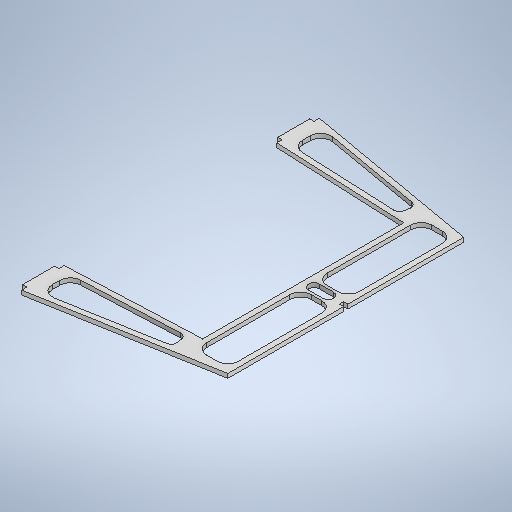
# Autodesk Inventor part: crush zone
Saved by Autodesk Inventor 2025.2 (Build 292293000, 293)
## iProperties
Created: 2025-01-25
Part Number: crush zone
Material: Generic
Document SubType Name: Modeling
Designer: alex
Density: 1 g/cm^3
Appearance: Default
Author: alex
Autodesk Inventor part; units mm, degrees
ref_plane "YZ Plane" through (0, 0, 0) normal (1, 0, 0) x (0, 1, 0)
ref_plane "XZ Plane" through (0, 0, 0) normal (0, 1, 0) x (-1, 0, 0)
ref_plane "XY Plane" through (0, 0, 0) normal (0, 0, 1) x (1, 0, 0)
sketch "Sketch1" plane through (0, 0, 0) normal (0, 1, 0) x (-1, 0, 0)
  line L0 (0, 0) -> (0, -76.2)
  line L1 (0, -76.2) -> (-10.16, -76.2)
  line L2 (-10.16, -76.2) -> (-10.16, -88.9)
  line L3 (-10.16, -88.9) -> (-327.3578, -102.7492)
  line L4 (0, 0) -> (-10.16, 0)
  line L5 (-10.16, 0) -> (-10.16, 12.7)
  line L6 (-10.16, 12.7) -> (-428.9578, -61.1454)
  line L7 (-428.9578, -61.1454) -> (-428.9578, -342.9)
  line L8 (-428.9578, -342.9) -> (-327.3578, -342.9)
  line L9 (-327.3578, -342.9) -> (-327.3578, -102.7492)
  line L10 (-365.4578, -323.85) -> (-390.8578, -323.85)
  line L11 (-416.2578, -298.45) -> (-416.2578, -99.2454)
  line L12 (-390.8578, -73.8454) -> (-365.4578, -73.8454)
  line L13 (-340.0578, -99.2454) -> (-340.0578, -298.45)
  line L14 (-294.1616, -50.2731) -> (-65.3707, -9.931)
  line L15 (-35.56, -34.9452) -> (-35.56, -52.9817)
  line L16 (-59.8521, -78.3575) -> (-289.4473, -88.3818)
  arc A0 (-340.0578, -99.2454) -> (-365.4578, -73.8454) centre (-365.4578, -99.2454) ccw
  arc A1 (-390.8578, -73.8454) -> (-416.2578, -99.2454) centre (-390.8578, -99.2454) ccw
  arc A2 (-416.2578, -298.45) -> (-390.8578, -323.85) centre (-390.8578, -298.45) ccw
  arc A3 (-365.4578, -323.85) -> (-340.0578, -298.45) centre (-365.4578, -298.45) ccw
  arc A4 (-35.56, -34.9452) -> (-65.3707, -9.931) centre (-60.96, -34.9452) ccw
  arc A5 (-59.8521, -78.3575) -> (-35.56, -52.9817) centre (-60.96, -52.9817) ccw
  line L17 (0, -685.8) -> (0, -609.6)
  line L18 (0, -609.6) -> (-10.16, -609.6)
  line L19 (-10.16, -609.6) -> (-10.16, -596.9)
  line L20 (-10.16, -596.9) -> (-327.3578, -583.0508)
  line L21 (0, -685.8) -> (-10.16, -685.8)
  line L22 (-10.16, -685.8) -> (-10.16, -698.5)
  line L23 (-10.16, -698.5) -> (-428.9578, -624.6546)
  line L24 (-428.9578, -624.6546) -> (-428.9578, -342.9)
  line L25 (-327.3578, -342.9) -> (-327.3578, -583.0508)
  line L26 (-365.4578, -361.95) -> (-390.8578, -361.95)
  line L27 (-416.2578, -387.35) -> (-416.2578, -586.5546)
  line L28 (-390.8578, -611.9546) -> (-365.4578, -611.9546)
  line L29 (-340.0578, -586.5546) -> (-340.0578, -387.35)
  line L30 (-294.1616, -635.5269) -> (-65.3707, -675.869)
  line L31 (-35.56, -650.8548) -> (-35.56, -632.8183)
  line L32 (-59.8521, -607.4425) -> (-289.4473, -597.4182)
  arc A6 (-365.4578, -611.9546) -> (-340.0578, -586.5546) centre (-365.4578, -586.5546) ccw
  arc A7 (-416.2578, -586.5546) -> (-390.8578, -611.9546) centre (-390.8578, -586.5546) ccw
  arc A8 (-390.8578, -361.95) -> (-416.2578, -387.35) centre (-390.8578, -387.35) ccw
  arc A9 (-340.0578, -387.35) -> (-365.4578, -361.95) centre (-365.4578, -387.35) ccw
  arc A10 (-65.3707, -675.869) -> (-35.56, -650.8548) centre (-60.96, -650.8548) ccw
  arc A11 (-35.56, -632.8183) -> (-59.8521, -607.4425) centre (-60.96, -632.8183) ccw
  line L33 (-428.9578, -337.82) -> (-418.7978, -337.82)
  line L34 (-418.7978, -337.82) -> (-418.7978, -347.98)
  line L35 (-418.7978, -347.98) -> (-428.9578, -347.98)
  line L36 (-387.0478, -330.2) -> (-352.7578, -330.2)
  line L37 (-340.0578, -342.9) -> (-340.0578, -342.9)
  line L38 (-352.7578, -355.6) -> (-387.0478, -355.6)
  line L39 (-399.7478, -342.9) -> (-399.7478, -342.9)
  arc A12 (-340.0578, -342.9) -> (-352.7578, -330.2) centre (-352.7578, -342.9) ccw
  arc A13 (-352.7578, -355.6) -> (-340.0578, -342.9) centre (-352.7578, -342.9) ccw
  arc A14 (-399.7478, -342.9) -> (-387.0478, -355.6) centre (-387.0478, -342.9) ccw
  arc A15 (-387.0478, -330.2) -> (-399.7478, -342.9) centre (-387.0478, -342.9) ccw
  line L40 (-304.5132, -64.681) -> (-302.5582, -77.5949)
  arc A16 (-294.1616, -50.2731) -> (-304.5132, -64.681) centre (-291.9562, -62.7801) ccw
  arc A17 (-302.5582, -77.5949) -> (-289.4473, -88.3818) centre (-290.0013, -75.6939) ccw
  line L41 (-304.5132, -621.119) -> (-302.5582, -608.2051)
  arc A18 (-289.4473, -597.4182) -> (-302.5582, -608.2051) centre (-290.0013, -610.1061) ccw
  arc A19 (-304.5132, -621.119) -> (-294.1616, -635.5269) centre (-291.9562, -623.0199) ccw
  point P0 (-300.8499, -88.8797)
  point P1 (-306.3685, -52.4255)
  point P2 (-300.8499, -596.9203)
  point P3 (-306.3685, -633.3745)
  point P4 (-340.0578, -342.9)
  dimension "d0" = 76.2
  dimension "d1" = 10.16
  dimension "d2" = 12.7
  dimension "d3" = 317.5
  dimension "d4" = 92.5
  dimension "d5" = 12.7
  dimension "d6" = 80
  dimension "d8" = 266.7
  dimension "d9" = 101.6
  dimension "d10" = 10.16
  dimension "d11" = 12.7
  dimension "d12" = 12.7
  dimension "d13" = 19.05
  dimension "d14" = 12.7
  dimension "d15" = 25.4
  dimension "d16" = 12.7
  dimension "d17" = 12.7
  dimension "d18" = 25.4
  dimension "d20" = 25.4
  dimension "d21" = 10.16
  dimension "d22" = 5.08
  dimension "d23" = 10.16
  dimension "d26" = 6.35
  dimension "d27" = 6.35
  dimension "d28" = 12.7
  dimension "d29" = 19.05
  dimension "d30" = 12.7
  dimension "d32" = 12.7
  dimension "d33" = 12.7
  constraints: 84 end point, 40 point on circle, 28 symmetric about line, 28 tangent, 20 centre point, 9 equal radius, 9 perpendicular, 9 point on line, 6 parallel, 4 horizontal, 2 vertical, 6 other
  measures "d0" distance of L0.start L0.end
  measures "d1" distance of L0.end L1.end
  measures "d2" distance of L1.end L2.end
  measures "d3" distance of L2.end L3.end
  measures "d4" angle of L2 L3
  measures "d5" distance of L4.end L5.end
  measures "d6" angle of L6 L5
  measures "d8" distance between parallel lines of L1 L8
  measures "d9" distance between parallel lines of L9 L7
  measures "d10" distance of L0.start L4.end
  measures "d11" distance between parallel lines of L9 L13
  measures "d12" distance between parallel lines of L7 L11
  measures "d13" distance between parallel lines of L8 L10
  measures "d14" distance from line of L6.end L12
  measures "d15" radius of A0
  measures "d16" distance between parallel lines of L6 L14
  measures "d17" distance between parallel lines of L3 L16
  measures "d18" distance between parallel lines of L2 L15
  measures "d20" radius of A4
  measures "d21" distance of L33.start L33.end
  measures "d22" distance of L7.end L33.start
  measures "d23" distance of L33.end L34.end
  measures "d26" distance between parallel lines of L10 L36
  measures "d27" distance between parallel lines of L26 L38
  measures "d28" distance between parallel lines of L25 L37
  measures "d29" distance between parallel lines of L34 L39
  measures "d30" radius of A12
  measures "d32" radius of A16
  measures "d33" radius of A18
extrude "Extrusion1" add sketch "Sketch1" along normal blind 10.16 contours L0 L1 L2 L3 L9 L8 A12 L36 A15 L34 L33 L7 L6 L5 L4 | L25 L20 L19 L18 L17 L21 L22 L23 L24 L35 L34 L8 A14 L38 A13
body "Solid1"
